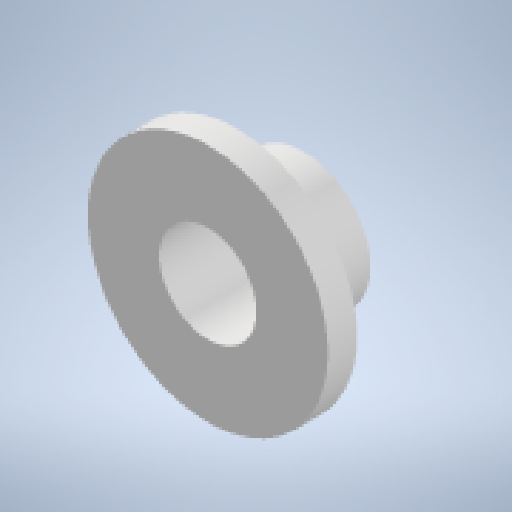
# Autodesk Inventor part: CAD_inner_3
Saved by Autodesk Inventor 2023 (Build 270158000, 158)
## iProperties
Created: 2023-04-09
Part Number: CAD_inner_3
Material: Generic
Document SubType Name: Modeling
Designer: steff
Density: 1 g/cm^3
Appearance: Default
Author: steff
## iProperties of the stored document CAD_inner_3DPrint.ipt
Created: 2023-04-10
Part Number: CAD_inner_3DPrint
Material: Generic
Document SubType Name: Modeling
Designer: steff
Density: 1 g/cm^3
Appearance: Default
Author: steff
Autodesk Inventor part; units mm, degrees
ref_plane "YZ Plane" through (0, 0, 0) normal (1, 0, 0) x (0, 1, 0)
ref_plane "XZ Plane" through (0, 0, 0) normal (0, 1, 0) x (-1, 0, 0)
ref_plane "XY Plane" through (0, 0, 0) normal (0, 0, 1) x (1, 0, 0)
sketch "Sketch1" plane through (0, 0, 0) normal (0, 0, 1) x (1, 0, 0)
  circle A0 centre (0, 0) radius 5.05
  circle A1 centre (0, 0) radius 6.9
  dimension "d0" = 10.1
  dimension "d1" = 13.8
  constraints: 2 centre point, 2 coincident
  measures "d0" diameter of A0
  measures "d1" diameter of A1
extrude "Extrusion1" add sketch "Sketch1" along normal blind 10
sketch "Sketch2" plane through (0, 0, 10) normal (0, 0, 1) x (1, 0, 0)
  circle A0 centre (0, 0) radius 12.5
  circle A1 centre (0, 0) radius 6.9 projected
  dimension "d4" = 25
  constraints: 1 centre point, 1 coincident
  measures "d4" diameter of A0
extrude "Extrusion2" add sketch "Sketch2" against normal blind 3
sketch "Sketch3" plane through (0, 0, 0) normal (0, 0, -1) x (-1, 0, 0)
  point P0 (0, 0)
sketch "Sketch4" plane through (0, 0, 0) normal (0, 0, -1) x (-1, 0, 0)
  point P0 (0, 0)
body "Solid1"
